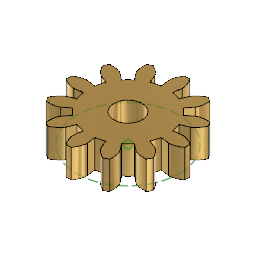
gear-encoder v1 (Autodesk Fusion 360 design; units mm, degrees)
description: Spur Gear; Module: 0.3; Num Teeth: 12; Pressure Angle: 20.0; Backlash: 0.00 mm
Autodesk Fusion 360 part; units mm, degrees
sketch "スケッチ1" plane through (0, 0, 0) normal (0, 0, 1) x (1, 0, 0) in component "Spur Gear (12 teeth)"
  circle A0 centre (0, 0) radius 1.3892
  circle A1 centre (0, 0) radius 0.5
extrude "押し出し1" add sketch "スケッチ1" along normal blind 1 in component "Spur Gear (12 teeth)"
sketch "スケッチ2" plane through (0, 0, 0) normal (0, 0, 1) x (1, 0, 0) in component "Spur Gear (12 teeth)"
  spline S0 degree 5 poles (1.6735, -0.2457) (1.6747, -0.2459) (1.677, -0.2462) (1.6806, -0.2466) (1.6853, -0.2468) (1.6912, -0.2468) (1.6972, -0.2467) (1.7032, -0.2464) (1.7091, -0.246) (1.7151, -0.2456) (1.7212, -0.2451) (1.7272, -0.2445) (1.7332, -0.2439) (1.7392, -0.2431) (1.7453, -0.2423) (1.7514, -0.2414) (1.7574, -0.2403) (1.7635, -0.2392) (1.7696, -0.2381) (1.7756, -0.2369) (1.7817, -0.2356) (1.7878, -0.2342) (1.7939, -0.2328) (1.8, -0.2313) (1.8061, -0.2298) (1.8122, -0.2282) (1.8183, -0.2265) (1.8244, -0.2248) (1.8306, -0.223) (1.8367, -0.2212) (1.8428, -0.2193) (1.8489, -0.2173) (1.855, -0.2153) (1.8611, -0.2132) (1.8673, -0.2111) (1.8734, -0.2089) (1.8795, -0.2067) (1.8856, -0.2044) (1.8917, -0.2021) (1.8979, -0.1997) (1.904, -0.1972) (1.9101, -0.1947) (1.9162, -0.1922) (1.9223, -0.1896) (1.9285, -0.1869) (1.9346, -0.1842) (1.9407, -0.1815) (1.9468, -0.1787) (1.9529, -0.1758) (1.959, -0.1729) (1.9651, -0.17) (1.9712, -0.167) (1.9773, -0.1639) (1.9833, -0.1608) (1.9894, -0.1577) (1.9955, -0.1545) (2.0016, -0.1512) (2.0076, -0.1479) (2.0137, -0.1446) (2.0198, -0.1412) (2.0258, -0.1378) (2.0319, -0.1343) (2.0379, -0.1308) (2.0439, -0.1272) (2.05, -0.1236) (2.056, -0.12) (2.062, -0.1163) (2.068, -0.1125) (2.074, -0.1087) (2.08, -0.1049) (2.086, -0.101) (2.0908, -0.0979) (2.0944, -0.0955) (2.0967, -0.0939) (2.0979, -0.0931) knots 0 0 0 0 0 0 0.01428571 0.02857143 0.04285714 0.05714286 0.07142857 0.08571429 0.1 0.11428571 0.12857143 0.14285714 0.15714286 0.17142857 0.18571429 0.2 0.21428571 0.22857143 0.24285714 0.25714286 0.27142857 0.28571429 0.3 0.31428571 0.32857143 0.34285714 0.35714286 0.37142857 0.38571429 0.4 0.41428571 0.42857143 0.44285714 0.45714286 0.47142857 0.48571429 0.5 0.51428571 0.52857143 0.54285714 0.55714286 0.57142857 0.58571429 0.6 0.61428571 0.62857143 0.64285714 0.65714286 0.67142857 0.68571429 0.7 0.71428571 0.72857143 0.74285714 0.75714286 0.77142857 0.78571429 0.8 0.81428571 0.82857143 0.84285714 0.85714286 0.87142857 0.88571429 0.9 0.91428571 0.92857143 0.94285714 0.95714286 0.97142857 0.98571429 1 1 1 1 1 1
  spline S1 degree 5 poles (1.6735, 0.2457) (1.6747, 0.2459) (1.677, 0.2462) (1.6806, 0.2466) (1.6853, 0.2468) (1.6912, 0.2468) (1.6972, 0.2467) (1.7032, 0.2464) (1.7091, 0.246) (1.7151, 0.2456) (1.7212, 0.2451) (1.7272, 0.2445) (1.7332, 0.2439) (1.7392, 0.2431) (1.7453, 0.2423) (1.7514, 0.2414) (1.7574, 0.2403) (1.7635, 0.2392) (1.7696, 0.2381) (1.7756, 0.2369) (1.7817, 0.2356) (1.7878, 0.2342) (1.7939, 0.2328) (1.8, 0.2313) (1.8061, 0.2298) (1.8122, 0.2282) (1.8183, 0.2265) (1.8244, 0.2248) (1.8306, 0.223) (1.8367, 0.2212) (1.8428, 0.2193) (1.8489, 0.2173) (1.855, 0.2153) (1.8611, 0.2132) (1.8673, 0.2111) (1.8734, 0.2089) (1.8795, 0.2067) (1.8856, 0.2044) (1.8917, 0.2021) (1.8979, 0.1997) (1.904, 0.1972) (1.9101, 0.1947) (1.9162, 0.1922) (1.9223, 0.1896) (1.9285, 0.1869) (1.9346, 0.1842) (1.9407, 0.1815) (1.9468, 0.1787) (1.9529, 0.1758) (1.959, 0.1729) (1.9651, 0.17) (1.9712, 0.167) (1.9773, 0.1639) (1.9833, 0.1608) (1.9894, 0.1577) (1.9955, 0.1545) (2.0016, 0.1512) (2.0076, 0.1479) (2.0137, 0.1446) (2.0198, 0.1412) (2.0258, 0.1378) (2.0319, 0.1343) (2.0379, 0.1308) (2.0439, 0.1272) (2.05, 0.1236) (2.056, 0.12) (2.062, 0.1163) (2.068, 0.1125) (2.074, 0.1087) (2.08, 0.1049) (2.086, 0.101) (2.0908, 0.0979) (2.0944, 0.0955) (2.0967, 0.0939) (2.0979, 0.0931) knots 0 0 0 0 0 0 0.01428571 0.02857143 0.04285714 0.05714286 0.07142857 0.08571429 0.1 0.11428571 0.12857143 0.14285714 0.15714286 0.17142857 0.18571429 0.2 0.21428571 0.22857143 0.24285714 0.25714286 0.27142857 0.28571429 0.3 0.31428571 0.32857143 0.34285714 0.35714286 0.37142857 0.38571429 0.4 0.41428571 0.42857143 0.44285714 0.45714286 0.47142857 0.48571429 0.5 0.51428571 0.52857143 0.54285714 0.55714286 0.57142857 0.58571429 0.6 0.61428571 0.62857143 0.64285714 0.65714286 0.67142857 0.68571429 0.7 0.71428571 0.72857143 0.74285714 0.75714286 0.77142857 0.78571429 0.8 0.81428571 0.82857143 0.84285714 0.85714286 0.87142857 0.88571429 0.9 0.91428571 0.92857143 0.94285714 0.95714286 0.97142857 0.98571429 1 1 1 1 1 1
  arc A0 (2.0979, -0.0931) -> (2.0979, 0.0931) centre (0, 0) ccw
  line L0 (1.3646, -0.2018) -> (1.6735, -0.2457)
  line L1 (1.3646, 0.2018) -> (1.6735, 0.2457)
  line L2 (1.3646, -0.2018) -> (1.3646, 0.2018)
extrude "押し出し2" add sketch "スケッチ2" along normal blind 1 in component "Spur Gear (12 teeth)"
pattern_circular "C パターン1" count 12 over 360 about axis through (0, 0, 0) along (0, 0, 1) of "押し出し2" in component "Spur Gear (12 teeth)"
sketch "スケッチ3" plane through (0, 0, 0) normal (0, 0, 1) x (1, 0, 0) in component "Spur Gear (12 teeth)"
  circle A0 centre (0, 0) radius 1.8 construction
component "Spur Gear (12 teeth)" placed x (1, 0, 0) y (0, 1, 0) z (0, 0, 1) at (0, 0, 0)
